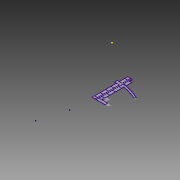
# Autodesk Inventor part: LabVIEWM0.5
Saved by Autodesk Inventor 2013 SP2 (Build 170200200, 200)
## iProperties
Created: 2014-11-17
Part Number: LabVIEWM0.5
Material: 常规
Document SubType Name: Modeling
Designer: 振胜
Density: 1 g/cm^3
Author: 振胜
Autodesk Inventor part; units mm, degrees
sketch "TEMP" plane through (0, 0, 0) normal (0, 0, 1) x (1, 0, 0)
  line L0 (1237.5395, -739.2114) -> (1240.1864, -734.0506) construction
  line L1 (1235.9851, -775.1327) -> (1263.1743, -787.8113)
  line L2 (1224.5874, -769.8179) -> (1235.9851, -775.1327)
  line L3 (1258.2688, -748.8776) -> (1250.0214, -745.0318) construction
  line L4 (1250.0214, -745.0318) -> (1237.5395, -739.2114)
  line L5 (1258.2688, -748.8776) -> (1237.5395, -739.2114) construction
  line L6 (1237.5395, -739.2114) -> (1240.1864, -734.0506)
  line L7 (1240.1864, -734.0506) -> (1226.8396, -727.205)
  line L8 (1240.1864, -734.0506) -> (1226.8396, -727.205) construction
  line L9 (1250.0214, -745.0318) -> (1277.2106, -757.7104)
  line L10 (1226.8396, -727.205) -> (1213.8396, -757.905)
  line L11 (1226.8396, -727.205) -> (1213.8396, -757.905) construction
  line L12 (1250.0214, -745.0318) -> (1235.9851, -775.1327)
  line L13 (1213.8396, -757.905) -> (1227.1864, -764.7506)
  line L14 (1213.8396, -757.905) -> (1227.1864, -764.7506) construction
  line L15 (1227.1864, -764.7506) -> (1224.5874, -769.8179)
  line L16 (1227.1864, -764.7506) -> (1224.5874, -769.8179) construction
  line L17 (1235.9851, -775.1327) -> (1244.2325, -778.9786) construction
  line L18 (1224.5874, -769.8179) -> (1244.2325, -778.9786) construction
  line L19 (1263.1743, -787.8113) -> (1277.2106, -757.7104)
  point P0 (1239.5055, -755.7006)
  dimension "d196" = 9.1
  dimension "d197" = 30
  dimension "d198" = 30
  measures "d196" distance of L5.start L3.end
  measures "d197" distance of L3.end L9.end
  measures "d198" distance of L12.end L1.end
sketch "TEMP2" plane through (0, 0, 0) normal (0, 0, 1) x (1, 0, 0)
  line L0 (1110, -1180.4746) -> (1113.8458, -1172.2272)
  line L1 (1068.2, -1174.6) -> (1110, -1180.4746)
  line L2 (1031.2, -1174.6) -> (1068.2, -1174.6)
  line L3 (1031.2, -1121.1) -> (1031.2, -1174.6)
  line L4 (1117.8, -1121.1) -> (1031.2, -1121.1)
  line L5 (1031.2, -1121.1) -> (1031.2, -1174.6) construction
  line L6 (1117.8, -1121.1) -> (1031.2, -1121.1) construction
  line L7 (1031.2, -1174.6) -> (1068.2, -1174.6) construction
  line L8 (1068.2, -1174.6) -> (1110, -1180.4746) construction
  line L9 (1110, -1180.4746) -> (1113.8458, -1172.2272) construction
  point P0 (1072.9976, -1158.9944)
sketch "TEMP3" plane through (0, 0, 0) normal (0, 0, 1) x (1, 0, 0)
  line L0 (1117.8, -1121.1) -> (1090.6108, -1108.4215) construction
  line L1 (1031.2, -1121.1) -> (1031.2, -1174.6) construction
  line L2 (1117.8, -1121.1) -> (1031.2, -1121.1) construction
  line L3 (1031.2, -1174.6) -> (1068.2, -1174.6) construction
  line L4 (1068.2, -1174.6) -> (1110, -1180.4746) construction
  line L5 (1110, -1180.4746) -> (1113.8458, -1172.2272) construction
  line L6 (1117.8, -1121.1) -> (1031.2, -1121.1)
  line L7 (1031.2, -1121.1) -> (1031.2, -1174.6)
  line L8 (1031.2, -1174.6) -> (1068.2, -1174.6)
  line L9 (1068.2, -1174.6) -> (1110, -1180.4746) construction
  line L10 (1110, -1180.4746) -> (1113.8458, -1172.2272) construction
  line L11 (1090.6108, -1108.4215) -> (1117.8, -1121.1) construction
  line L12 (1117.8, -1121.1) -> (1091.3363, -1177.8516)
  line L13 (1091.3363, -1177.8516) -> (1068.2, -1174.6)
  point P0 (1077.5926, -1151.6555)
ref_plane "工作平面1" through (0, 0, 0) normal (0, 0, 1) x (1, 0, 0)
sketch "草图1" plane through (0, 0, 0) normal (0, 0, 1) x (1, 0, 0)
  line L0 (727.5, -616.2) -> (727.5, -673.6)
  line L1 (727.5, -616.2) -> (765.5, -616.2)
  line L2 (765.5, -616.2) -> (825.5, -616.2)
  line L3 (765.5, -616.2) -> (765.5, -504.2)
  line L4 (765.5, -504.2) -> (765.5, -444.2)
  line L5 (765.5, -444.2) -> (825.5, -444.2)
  line L6 (825.5, -444.2) -> (825.5, -504.2)
  line L7 (825.5, -504.2) -> (825.5, -616.2)
  line L8 (825.5, -504.2) -> (765.5, -504.2)
  line L9 (825.5, -444.2) -> (849.2, -444.2)
  line L10 (849.2, -444.2) -> (849.2, -450.2)
  line L11 (849.2, -450.2) -> (868.2, -450.2)
  line L12 (868.2, -450.2) -> (868.2, -502.2)
  line L13 (868.2, -502.2) -> (849.2, -502.2)
  line L14 (849.2, -502.2) -> (849.2, -450.2)
  line L15 (849.2, -502.2) -> (849.2, -506.7)
  line L16 (849.2, -506.7) -> (909.2, -506.7)
  line L17 (909.2, -506.7) -> (909.2, -613.1)
  line L18 (909.2, -613.1) -> (849.2, -613.1)
  line L19 (849.2, -613.1) -> (849.2, -506.7)
  line L20 (727.5, -673.6) -> (765.5, -673.6)
  line L21 (765.5, -673.6) -> (765.5, -786.6)
  line L22 (765.5, -786.6) -> (825.5, -786.6)
  line L23 (825.5, -786.6) -> (825.5, -673.6)
  line L24 (825.5, -673.6) -> (765.5, -673.6)
  line L25 (765.5, -786.6) -> (765.5, -897.6)
  line L26 (765.5, -897.6) -> (825.5, -897.6)
  line L27 (825.5, -897.6) -> (825.5, -786.6)
  line L28 (765.5, -897.6) -> (765.5, -1008.6)
  line L29 (765.5, -1008.6) -> (825.5, -1008.6)
  line L30 (825.5, -1008.6) -> (825.5, -897.6)
  line L31 (765.5, -1008.6) -> (765.5, -1125.1)
  line L32 (765.5, -1125.1) -> (825.5, -1125.1)
  line L33 (825.5, -1125.1) -> (825.5, -1008.6)
  line L34 (765.5, -1125.1) -> (765.5, -1174.6) construction
  line L35 (765.5, -1174.6) -> (825.5, -1174.6)
  line L36 (825.5, -1174.6) -> (825.5, -1125.1)
  line L37 (825.5, -1174.6) -> (849.2, -1174.6)
  line L38 (849.2, -613.1) -> (849.2, -623.1)
  line L39 (849.2, -623.1) -> (916.2, -623.1)
  line L40 (916.2, -623.1) -> (916.2, -626.6)
  line L41 (849.2, -623.1) -> (849.2, -668.1)
  line L42 (849.2, -668.1) -> (916.2, -668.1) construction
  line L43 (916.2, -668.1) -> (916.2, -664.6)
  line L44 (849.2, -668.1) -> (849.2, -681.1)
  line L45 (849.2, -681.1) -> (849.2, -1050.1)
  line L46 (849.2, -1050.1) -> (909.2, -1050.1) construction
  line L47 (909.2, -1050.1) -> (909.2, -1091.6)
  line L48 (909.2, -1091.6) -> (909.2, -1121.1)
  line L49 (909.2, -1121.1) -> (849.2, -1121.1)
  line L50 (849.2, -1121.1) -> (849.2, -1050.1)
  line L51 (909.2, -1091.6) -> (849.2, -1091.6) construction
  line L52 (849.2, -1174.6) -> (849.2, -1121.1)
  line L53 (849.2, -1174.6) -> (1031.2, -1174.6)
  line L54 (1031.2, -1121.1) -> (909.2, -1121.1)
  line L55 (916.2, -626.6) -> (1226.4, -727) construction
  arc A0 (1226.4, -727) -> (916.2, -626.6) centre (761.993, -1632.4479) ccw
  line L56 (916.2, -664.6) -> (1213.4, -757.7) construction
  arc A1 (1213.4, -757.7) -> (916.2, -664.6) centre (605.6007, -2177.0365) ccw
  line L57 (916.2, -668.1) -> (909.2, -668.1)
  line L58 (909.2, -613.1) -> (909.2, -668.1) construction
  line L59 (909.2, -668.1) -> (909.2, -710.2)
  line L60 (909.2, -710.2) -> (849.2, -710.2)
  line L61 (909.2, -710.2) -> (909.2, -841.8)
  line L62 (909.2, -841.8) -> (849.2, -841.8)
  line L63 (909.2, -841.8) -> (909.2, -953.1)
  line L64 (909.2, -953.1) -> (909.2, -1064)
  line L65 (909.2, -1064) -> (849.2, -1064)
  line L66 (909.2, -953.1) -> (849.2, -953.1)
  line L67 (765.5, -1174.6) -> (761.5, -1174.6)
  line L68 (761.5, -1174.6) -> (761.5, -1125.1)
  line L69 (761.5, -1125.1) -> (765.5, -1125.1)
  line L70 (1213.4, -757.7) -> (1226.4, -727)
  line L71 (1031.2, -1121.1) -> (1031.2, -1174.6)
  point P0 (0, 0)
  dimension "d89" = 38
  dimension "d90" = 60
  dimension "d91" = 112
  dimension "d92" = 60
  dimension "d93" = 60
  dimension "d94" = 23.7
  dimension "d95" = 6
  dimension "d96" = 19
  dimension "d97" = 52
  dimension "d98" = 4.5
  dimension "d99" = 60
  dimension "d101" = 106.4
  dimension "d103" = 113
  dimension "d104" = 60
  dimension "d105" = 111
  dimension "d106" = 111
  dimension "d107" = 60
  dimension "d108" = 116.5
  dimension "d109" = 60
  dimension "d110" = 49.5
  dimension "d111" = 23.7
  dimension "d112" = 10
  dimension "d113" = 67
  dimension "d114" = 3.5
  dimension "d115" = 45
  dimension "d116" = 3.5
  dimension "d117" = 13
  dimension "d118" = 369
  dimension "d119" = 60
  dimension "d120" = 41.5
  dimension "d121" = 29.5
  dimension "d122" = 182
  dimension "d123" = 100.4
  dimension "d124" = 310.2
  dimension "d125" = 1017.6
  dimension "d126" = 93.1
  dimension "d127" = 297.2
  dimension "d128" = 1544
  dimension "d184" = 53.5
  dimension "d185" = 314.0223
  dimension "d186" = 360.3281
  dimension "d187" = 435.0585
  dimension "d189" = 42.1
  dimension "d190" = 131.6
  dimension "d191" = 111.3
  dimension "d192" = 110.9
  dimension "d193" = 4
  constraints: 145 end point, 39 perpendicular, 15 parallel, 10 point on line, 6 collinear, 4 point on circle, 2 centre point, 1 vertical
  measures "d89" distance of L0.start L1.end
  measures "d90" distance of L1.end L2.end
  measures "d91" distance of L1.end L3.end
  measures "d92" distance of L3.end L4.end
  measures "d93" distance of L4.end L5.end
  measures "d94" distance of L5.end L9.end
  measures "d95" distance of L9.end L10.end
  measures "d96" distance of L10.end L11.end
  measures "d97" distance of L11.end L12.end
  measures "d98" distance of L13.end L15.end
  measures "d99" distance of L15.end L16.end
  measures "d101" distance of L16.end L17.end
  measures "d103" distance of L20.end L21.end
  measures "d104" distance of L21.end L22.end
  measures "d105" distance of L21.end L25.end
  measures "d106" distance of L25.end L28.end
  measures "d107" distance of L28.end L29.end
  measures "d108" distance of L28.end L31.end
  measures "d109" distance of L31.end L32.end
  measures "d110" distance of L31.end L34.end
  measures "d111" distance of L35.end L37.end
  measures "d112" distance of L18.end L38.end
  measures "d113" distance of L38.end L39.end
  measures "d114" distance of L39.end L40.end
  measures "d115" distance of L38.end L41.end
  measures "d116" distance of L42.end L43.end
  measures "d117" distance of L41.end L44.end
  measures "d118" distance of L44.end L45.end
  measures "d119" distance of L45.end L46.end
  measures "d120" distance of L46.end L47.end
  measures "d121" distance of L47.end L48.end
  measures "d122" distance of L37.end L53.end
  measures "d123" vertical distance of L40.end L55.end
  measures "d124" horizontal distance of L55.end L40.end
  measures "d125" radius of A0
  measures "d126" vertical distance of L56.end L43.end
  measures "d127" horizontal distance of L56.end L43.end
  measures "d128" radius of A1
  measures "d184" distance between parallel lines of L54 L37
  measures "d185" distance from line of point (0, 0) L55
  measures "d186" distance from line of point (0, 0) L56
  measures "d187" distance from line of L54.start L55
  measures "d189" distance of L57.end L59.end
  measures "d190" distance of L59.end L61.end
  measures "d191" distance of L61.end L63.end
  measures "d192" distance of L63.end L64.end
  measures "d193" distance of L34.end L67.end
extrude "拉伸1" add sketch "草图1" against normal blind 1
sketch "草图2" plane through (0, 0, 0) normal (0, 0, 1) x (1, 0, 0)
  line L0 (1213.4, -757.7) -> (1226.4, -727) construction
  arc A0 (1226.4, -727) -> (916.2, -626.6) centre (761.993, -1632.4479) ccw construction
  arc A1 (1213.4, -757.7) -> (916.2, -664.6) centre (605.6007, -2177.0365) ccw construction
  line L1 (1237.0998, -739.0064) -> (1239.7468, -733.8456) construction
  line L2 (1235.5455, -774.9277) -> (1262.7347, -787.6063)
  line L3 (1224.1478, -769.6129) -> (1235.5455, -774.9277)
  line L4 (1257.8292, -748.6726) -> (1249.5818, -744.8268) construction
  line L5 (1249.5818, -744.8268) -> (1237.0998, -739.0064)
  line L6 (1257.8292, -748.6726) -> (1237.0998, -739.0064) construction
  line L7 (1237.0998, -739.0064) -> (1239.7468, -733.8456)
  line L8 (1239.7468, -733.8456) -> (1226.4, -727)
  line L9 (1239.7468, -733.8456) -> (1226.4, -727) construction
  line L10 (1249.5818, -744.8268) -> (1276.771, -757.5054)
  line L11 (1226.4, -727) -> (1213.4, -757.7)
  line L12 (1226.4, -727) -> (1213.4, -757.7) construction
  line L13 (1249.5818, -744.8268) -> (1235.5455, -774.9277)
  line L14 (1213.4, -757.7) -> (1226.7468, -764.5456)
  line L15 (1213.4, -757.7) -> (1226.7468, -764.5456) construction
  line L16 (1226.7468, -764.5456) -> (1224.1478, -769.6129)
  line L17 (1226.7468, -764.5456) -> (1224.1478, -769.6129) construction
  line L18 (1235.5455, -774.9277) -> (1243.7929, -778.7736) construction
  line L19 (1224.1478, -769.6129) -> (1243.7929, -778.7736) construction
  line L20 (1262.7347, -787.6063) -> (1276.771, -757.5054)
  point P0 (0, 0)
  constraints: 2 other
extrude "拉伸2" add sketch "草图2" against normal blind 1 contours L3 L16 L14 L11 L8 L7 L5 L13
sketch "草图3" plane through (1224.1478, -769.6129, -1) normal (-0.4226183, -0.9063078, 0) x (0.9063078, -0.4226183, 0)
  line L0 (12.576, 1) -> (12.576, 0) construction
  line L1 (12.576, 0.5) -> (42.576, 15.5)
  line L2 (12.576, 1) -> (42.576, 16)
  line L3 (42.576, 16) -> (42.576, 15.5)
  line L4 (12.576, 1) -> (12.576, 0.5)
  point P0 (-1434.7071, 1)
  dimension "d201" = 15
  dimension "d203" = 30
  constraints: 8 end point, 1 collinear, 1 midpoint, 1 parallel, 1 vertical
  measures "d201" vertical distance of L1.start L1.end
  measures "d203" horizontal distance of L1.start L1.end
extrude "拉伸3" add sketch "草图3" against normal up to surface (33.2127 mm away)
ref_plane "工作平面2" through (999.7, -1174.6, 0) normal (1, 0, 0) x (0, 0, -1)
sketch "草图4" plane through (999.7, -1174.6, 0) normal (1, 0, 0) x (0, 0, -1)
  line L0 (0, 53.5) -> (1, 53.5) construction
  line L1 (0.5, 53.5) -> (-20.5, 95.5)
  line L2 (0.5, 53.5) -> (0.1, 53.5)
  line L3 (0.1, 53.5) -> (-20.9, 95.5)
  line L4 (-20.9, 95.5) -> (-20.5, 95.5)
  line L5 (-20.9, 95.5) -> (-20.9, 122.5)
  line L6 (-20.9, 122.5) -> (-20.5, 122.5)
  line L7 (-20.5, 122.5) -> (-20.5, 95.5)
  point P0 (0, 1174.6)
  dimension "d207" = 21
  dimension "d209" = 42
  dimension "d210" = 0.4
  dimension "d211" = 27
  dimension "d212" = 0.4
  constraints: 14 end point, 2 parallel, 2 perpendicular, 1 midpoint, 1 point on line
  measures "d207" horizontal distance of L1.start L1.end
  measures "d209" vertical distance of L1.start L1.end
  measures "d210" distance of L1.start L2.end
  measures "d211" distance of L3.end L5.end
  measures "d212" distance of L5.end L6.end
extrude "拉伸4" add sketch "草图4" against normal blind 42
sketch "草图5" plane through (999.7, -1174.6, 0) normal (1, 0, 0) x (0, 0, -1)
  line L0 (-20.5, 122.5) -> (-20.9, 122.5) construction
  line L1 (-20.9, 122.5) -> (-20.9, 95.5) construction
  line L2 (-20.5, 95.5) -> (-20.5, 122.5) construction
  line L3 (-20.5, 122.5) -> (-20.9, 122.5)
  line L4 (-20.9, 122.5) -> (-20.9, 95.5)
  line L5 (-20.9, 95.5) -> (-20.5, 95.5)
  line L6 (-20.5, 95.5) -> (-20.5, 122.5)
  line L7 (-20.5, 95.5) -> (-41.5, 53.5)
  line L8 (-20.9, 95.5) -> (-41.9, 53.5)
  line L9 (-41.9, 53.5) -> (-41.5, 53.5)
  point P0 (0, 1174.6)
  dimension "d215" = 42
  dimension "d217" = 21
  constraints: 14 end point, 3 parallel, 2 horizontal, 1 perpendicular
  measures "d215" vertical distance of L5.end L7.end
  measures "d217" horizontal distance of L5.end L7.end
extrude "拉伸5" add sketch "草图5" along normal blind 18
ref_plane "工作平面3" through (978.7, -1174.6, 0) normal (-1, 0, 0) x (0, 0, 1)
mirror "镜像1" about plane through (978.7, -1174.6, 0) normal (-1, 0, 0) of "拉伸5"
sketch "草图6" plane through (0, 0, 0) normal (0, 0, 1) x (1, 0, 0)
  line L0 (1031.2, -1174.6) -> (1031.2, -1121.1) construction
  line L1 (1117.8, -1121.1) -> (1090.6108, -1108.4215) construction
  line L2 (1031.2, -1121.1) -> (1031.2, -1174.6) construction
  line L3 (1117.8, -1121.1) -> (1031.2, -1121.1) construction
  line L4 (1031.2, -1174.6) -> (1068.2, -1174.6) construction
  line L5 (1068.2, -1174.6) -> (1110, -1180.4746) construction
  line L6 (1110, -1180.4746) -> (1113.8458, -1172.2272) construction
  line L7 (1117.8, -1121.1) -> (1031.2, -1121.1)
  line L8 (1031.2, -1121.1) -> (1031.2, -1174.6)
  line L9 (1031.2, -1174.6) -> (1068.2, -1174.6)
  line L10 (1068.2, -1174.6) -> (1110, -1180.4746) construction
  line L11 (1110, -1180.4746) -> (1113.8458, -1172.2272) construction
  line L12 (1090.6108, -1108.4215) -> (1117.8, -1121.1) construction
  line L13 (1117.8, -1121.1) -> (1091.3363, -1177.8516)
  line L14 (1091.3363, -1177.8516) -> (1068.2, -1174.6)
  point P0 (0, 0)
  constraints: 2 other
extrude "拉伸6" add sketch "草图6" against normal blind 1
ref_plane "工作平面5" through (1109.1363, -1139.6793, 0) normal (-0.4226183, -0.9063078, 0) x (0.9063078, -0.4226183, 0)
ref_plane "工作平面4" through (1117.8, -1121.1, 0) normal (-0.4226183, -0.9063078, 0) x (0.9063078, -0.4226183, 0)
sketch "草图8" plane through (1109.1363, -1139.6793, 0) normal (-0.4226183, -0.9063078, 0) x (0.9063078, -0.4226183, 0)
  line L0 (0, 0) -> (0, -1) construction
  line L1 (0, 0) -> (-30, 0) construction
  line L2 (-30, 0) -> (-30, -1) construction
  line L3 (-30, -0.5) -> (0, 14.5)
  line L4 (-30, -0.5) -> (-30, -0.1)
  line L5 (-30, -0.1) -> (0, 14.9)
  line L6 (0, 14.9) -> (0, 14.5)
  point P0 (-1486.8682, 0)
  dimension "d223" = 30
  dimension "d224" = 30
  dimension "d225" = 15
  dimension "d226" = 1
  dimension "d227" = 0.4
  constraints: 12 end point, 2 perpendicular, 1 midpoint, 1 parallel, 1 point on line, 1 vertical
  measures "d223" distance of L0.start L1.end
  measures "d224" horizontal distance of L3.start L3.end
  measures "d225" vertical distance of L3.start L3.end
  measures "d226" distance of L1.end L2.end
  measures "d227" distance of L3.start L4.end
extrude "拉伸7" add sketch "草图8" along normal blind 15
